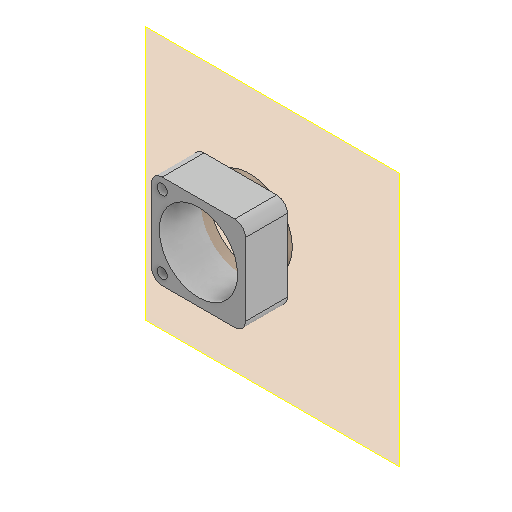
# Autodesk Inventor part: 30_Cube_SQUID_Z_Focus_spacer_v3
Saved by Autodesk Inventor 2022 (Build 260153000, 153)
## iProperties
Created: 2022-03-03
Part Number: 30_Cube_SQUID_Z_Focus_spacer_v3
Material: Generic
Document SubType Name: Modeling
Designer: Prakash Lab
Density: 1 g/cm^3
Appearance: Default
Author: Prakash Lab
Autodesk Inventor part; units mm, degrees
ref_plane "YZ Plane" through (0, 0, 0) normal (1, 0, 0) x (0, 1, 0)
ref_plane "XZ Plane" through (0, 0, 0) normal (0, 1, 0) x (-1, 0, 0)
ref_plane "XY Plane" through (0, 0, 0) normal (0, 0, 1) x (1, 0, 0)
ref_plane "Work Plane1" through (0, 0, 0) normal (0, 0, 1) x (1, 0, 0)
sketch "Sketch1" plane through (0, 0, 0) normal (0, 0, 1) x (1, 0, 0)
  line L0 (3.99, 16.87) -> (-0.09, 16.87) projected
  line L1 (-3.99, 20.77) -> (-0.09, 16.87) projected
  line L2 (-3.99, 24.85) -> (-3.99, 20.77) projected
  line L3 (-37.73, 24.85) -> (-3.99, 24.85) projected
  line L4 (-37.73, 16.87) -> (-37.73, 24.85) projected
  line L5 (-45.71, 16.87) -> (-37.73, 16.87) projected
  line L6 (-45.71, -16.87) -> (-45.71, -13.8689) projected
  line L7 (-41.63, -16.87) -> (-45.71, -16.87) projected
  line L8 (-37.73, -20.77) -> (-41.63, -16.87) projected
  line L9 (-37.73, -20.77) -> (-37.73, -24.85) projected
  line L10 (-37.73, -24.85) -> (-3.99, -24.85) projected
  line L11 (-3.99, -24.85) -> (-3.99, -20.77) projected
  line L12 (-0.09, -16.87) -> (-3.99, -20.77) projected
  line L13 (-0.09, -16.87) -> (3.99, -16.87) projected
  line L14 (3.99, -16.87) -> (3.99, 16.87) projected
  arc A0 (-35.53, 10.1) -> (-37.83, 7.8) centre (-35.53, 7.8) ccw projected
  line L15 (-37.83, -16.97) -> (-37.83, 16.97) construction
  arc A1 (-37.83, -7.8) -> (-35.53, -10.1) centre (-35.53, -7.8) ccw projected
  arc A2 (-19.93, -10.1) -> (-17.63, -7.8) centre (-19.93, -7.8) ccw projected
  arc A3 (-17.63, 7.8) -> (-19.93, 10.1) centre (-19.93, 7.8) ccw projected
  line L16 (-37.83, -7.8) -> (-37.83, 7.8)
  line L17 (-35.53, 10.1) -> (-19.93, 10.1)
  line L18 (-17.63, 7.8) -> (-17.63, -7.8)
  line L19 (-35.53, -10.1) -> (-19.93, -10.1)
  circle A4 centre (-27.73, 0) radius 8.4
  line L20 (-45.71, 13.8689) -> (-40.3869, 13.8689) projected
  line L21 (-40.3869, 13.8689) -> (-34.7289, 19.5269) projected
  line L22 (-34.7289, 19.5269) -> (-8.86, 19.5269) projected
  line L23 (-8.86, 19.5269) -> (-8.86, -19.5269) projected
  line L24 (-8.86, -19.5269) -> (-34.7289, -19.5269) projected
  line L25 (-34.7289, -19.5269) -> (-40.3869, -13.8689) projected
  line L26 (-40.3869, -13.8689) -> (-45.71, -13.8689) projected
  line L27 (-45.71, 13.8689) -> (-45.71, 16.87) projected
  point P0 (0, 0)
  point P1 (-17.63, -7.8)
  constraints: 8 end point, 2 perpendicular, 1 centre point, 1 collinear, 1 tangent, 1 vertical
extrude "Extrusion1" add sketch "Sketch1" along normal blind 9 contours L17 A3 L18 A2 L19 A1 L16 A0
sketch "Sketch2" plane through (0, 0, 9) normal (0, 0, 1) x (1, 0, 0)
  circle A0 centre (-20.86, 0) radius 16.97 construction
  line L0 (-19.93, 10.1) -> (-35.53, 10.1) projected
  arc A1 (-35.53, 10.1) -> (-37.83, 7.8) centre (-35.53, 7.8) ccw projected
  line L1 (-37.83, 7.8) -> (-37.83, -7.8) projected
  arc A2 (-37.83, -7.8) -> (-35.53, -10.1) centre (-35.53, -7.8) ccw projected
  line L2 (-35.53, -10.1) -> (-19.93, -10.1) projected
  arc A3 (-19.93, -10.1) -> (-17.63, -7.8) centre (-19.93, -7.8) ccw projected
  line L3 (-17.63, -7.8) -> (-17.63, 7.8) projected
  arc A4 (-17.63, 7.8) -> (-19.93, 10.1) centre (-19.93, 7.8) ccw projected
  point P0 (0, 0)
hole "Hole1" at (-35.53, -7.8, 9) at (-35.53, 7.8, 9) direction (0, 0, -1) diameter 2.2 depth 15 tip angle 118
sketch "Sketch3" plane through (0, 0, 0) normal (0, 0, -1) x (-1, 0, 0)
  circle A0 centre (27.73, 0) radius 8.4 projected
  circle A1 centre (27.73, 0) radius 9.25 projected
  circle A2 centre (27.73, 0) radius 9.15
  point P0 (0, 0)
  dimension "d10" = 0.1
  constraints: 1 centre point
  measures "d10" radial gap between concentric circles of A1 A2
extrude "Extrusion2" add sketch "Sketch3" along normal blind 2 contours A2
body "Solid1"
